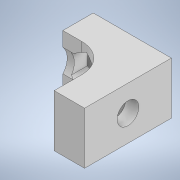
# Autodesk Inventor part: Soporte Cajas
Saved by Autodesk Inventor 2020 (Build 240168000, 168)
## iProperties
Created: 2021-01-15
Part Number: Soporte Cajas
Material: Generic
Document SubType Name: Modeling
Designer: Carlos
Density: 1 g/cm^3
Appearance: Default
Author: Carlos
Autodesk Inventor part; units mm, degrees
ref_plane "YZ Plane" through (0, 0, 0) normal (1, 0, 0) x (0, 1, 0)
ref_plane "XZ Plane" through (0, 0, 0) normal (0, 1, 0) x (-1, 0, 0)
sketch "Sketch1" plane through (0, 0, 0) normal (0, 1, 0) x (-1, 0, 0)
  line L0 (0, 0) -> (18, 0)
  line L1 (0, 0) -> (0, 20)
  line L2 (18, 0) -> (18, 7)
  line L3 (0, 20) -> (7, 20)
  line L4 (7, 20) -> (7, 7)
  line L5 (7, 7) -> (18, 7)
  dimension "d0" = 18
  dimension "d1" = 20
  dimension "d2" = 7
  dimension "d3" = 7
  constraints: 12 end point, 2 horizontal, 2 perpendicular, 2 vertical
  measures "d0" distance of L0.start L0.end
  measures "d1" distance of L0.start L1.end
  measures "d2" distance of L0.end L2.end
  measures "d3" distance of L1.end L3.end
extrude "Extrusion1" add sketch "Sketch1" along normal blind 12
sketch "Sketch3" plane through (-18, 0, 7) normal (0, 0, 1) x (1, 0, 0)
  line L0 (0, 0) -> (11, 0) projected
  line L1 (11, 12) -> (18, 12) projected
  line L2 (0, 0) -> (11, 0)
  line L3 (11, 0) -> (11, 12)
  line L4 (11, 12) -> (0, 12)
  line L5 (0, 12) -> (0, 0)
  circle A0 centre (5.5, 6) radius 2.5
  line L6 (5.5, 6) -> (0, 6)
  line L7 (0, 0) -> (0, 12) projected
  point P0 (18, 0)
  dimension "d7" = 5
  dimension "d24" = 5.5
  constraints: 10 end point, 2 parallel, 1 centre point, 1 horizontal, 1 midpoint, 1 perpendicular
  measures "d7" diameter of A0
  measures "d24" distance of L6.start L6.end
extrude "Extrusion2" cut sketch "Sketch3" against normal through all contours A0
sketch "Sketch4" plane through (-18, 0, 7) normal (0, 0, 1) x (1, 0, 0)
  circle A0 centre (5.5, 6) radius 2.5 projected
  line L0 (5.5, 10.4456) -> (9.35, 8.2228)
  line L1 (9.35, 8.2228) -> (9.35, 3.7772)
  line L2 (9.35, 3.7772) -> (5.5, 1.5544)
  line L3 (5.5, 1.5544) -> (1.65, 3.7772)
  line L4 (1.65, 3.7772) -> (1.65, 8.2228)
  line L5 (1.65, 8.2228) -> (5.5, 10.4456)
  line L6 (0, 0) -> (0, 12) projected
  point P0 (18, 0)
  dimension "d10" = 7.7
  dimension "d21" = 1.65
  constraints: 12 end point, 1 coincident, 13 other
  measures "d10" distance between parallel lines of L1 L4
  measures "d21" distance between parallel lines of L6 L4
extrude "Extrusion3" cut sketch "Sketch4" against normal blind 4
sketch "Sketch5" plane through (0, 0, 20) normal (1, 0, 0) x (0, 0, -1)
  line L0 (0, 0) -> (0, 12) projected
  line L1 (20, 0) -> (20, 12) projected
  line L2 (0, 0) -> (20, 0)
  line L3 (20, 0) -> (20, 12)
  line L4 (20, 12) -> (0, 12)
  line L5 (0, 12) -> (0, 0)
  circle A0 centre (10, 6) radius 2.5
  dimension "d13" = 5
  constraints: 8 end point, 2 parallel, 1 centre point, 1 horizontal, 1 perpendicular
  measures "d13" diameter of A0
extrude "Extrusion4" cut sketch "Sketch5" against normal through all contours A0
sketch "Sketch6" plane through (-7, 0, 7) normal (-1, 0, 0) x (0, 0, 1)
  circle A0 centre (3, 6) radius 2.5 projected
  circle A1 centre (3, 6) radius 4
  point P0 (-7, 0)
  dimension "d16" = 8
  constraints: 1 centre point, 1 coincident
  measures "d16" diameter of A1
extrude "Extrusion5" cut sketch "Sketch6" along normal blind 13 and the other way blind 4
fillet "Fillet1" radius 6.6 2 edges at (-7, 10.3229, 7) (-7, 1.6771, 7)
ref_plane "Work Plane1" through (0, 6, 0) normal (0, 1, 0) x (1, 0, 0)
sketch "Sketch7" plane through (0, 6, 0) normal (0, 1, 0) x (1, 0, 0)
  line L0 (-15, 0) -> (-10, 0) projected
  line L1 (-12.5, 0) -> (-9, 0)
  line L2 (0, 0) -> (-18, 0) projected
  circle A0 centre (-9, 0) radius 0.5
  line L3 (-12.5, 0) -> (-12.5, -3)
  line L4 (-15, -3) -> (-10, -3) projected
  dimension "d26" = 3.5
  dimension "d27" = 1
  constraints: 4 end point, 3 midpoint, 1 centre point, 1 coincident
  measures "d26" distance of L1.start L1.end
  measures "d27" diameter of A0
revolve "Revolution1" cut sketch "Sketch7" angle 360 about axis through (-12.5, 6, 0) along (0, 0, 1)
body "Solid1"
